Autodesk Fusion 360 part; units mm, degrees
(part 2 of 5)
sketch "Sketch8" plane through (0, 0, 0) normal (0, -1, 0) x (1, 0, 0)
  line L0 (30.55, -4) -> (30.55, 20)
  line L1 (30.55, 20) -> (28.55, 20)
  line L2 (28.55, 20) -> (28.55, -4)
  line L3 (30.55, 20) -> (28.55, 20)
  line L4 (30.55, 36.5) -> (30.55, 20)
  line L5 (-30.55, 20) -> (-28.55, 20)
  line L6 (-30.55, 36.5) -> (-30.55, 20)
  line L7 (28.55, 20) -> (-28.55, 20)
  line L8 (-19.3, 36.5) -> (-19.3, 34.25)
  line L9 (-24.3, 29.25) -> (-26.05, 29.25)
  line L10 (19.3, 36.5) -> (19.3, 34.25)
  line L11 (24.3, 29.25) -> (26.05, 29.25)
  line L12 (-28.55, 26.75) -> (-28.55, 20)
  line L13 (28.55, 26.75) -> (28.55, 20)
  line L14 (-28.05, 39) -> (-21.8, 39)
  line L15 (21.8, 39) -> (28.05, 39)
  arc A0 (30.55, 36.5) -> (28.05, 39) centre (28.05, 36.5) ccw
  arc A1 (-28.05, 39) -> (-30.55, 36.5) centre (-28.05, 36.5) ccw
  arc A2 (21.8, 39) -> (19.3, 36.5) centre (21.8, 36.5) ccw
  arc A3 (28.55, 26.75) -> (26.05, 29.25) centre (26.05, 26.75) ccw
  arc A4 (-26.05, 29.25) -> (-28.55, 26.75) centre (-26.05, 26.75) ccw
  arc A5 (-19.3, 36.5) -> (-21.8, 39) centre (-21.8, 36.5) ccw
  arc A6 (19.3, 34.25) -> (24.3, 29.25) centre (24.3, 34.25) ccw
  arc A7 (-24.3, 29.25) -> (-19.3, 34.25) centre (-24.3, 34.25) ccw
  line L16 (28.55, -4) -> (30.55, -4)
  point P0 (-30.55, 39)
  point P1 (-19.3, 39)
  point P2 (-19.3, 29.25)
  point P3 (-28.55, 29.25)
  point P4 (19.3, 39)
  point P5 (19.3, 29.25)
  point P6 (28.55, 29.25)
  dimension "d41" = 61.1
  dimension "d51" = 9.75
  dimension "d52" = 9.75
  dimension "d53" = 9.25
  dimension "d54" = 9.25
  dimension "d55" = 11.25
  dimension "d56" = 9.25
  dimension "d57" = 2.5
  dimension "d58" = 2.5
  dimension "d59" = 5
  constraint horizontal L3
  constraint vertical L4
  constraint coincident L0.end L1.start
  constraint horizontal L5
  constraint vertical L6
  constraint horizontal L0.end L5.start
  constraint vertical L8
  constraint horizontal L9
  constraint vertical L10
  constraint horizontal L11
  constraint perpendicular L7 L12
  constraint coincident L1.end L2.start
  constraint perpendicular L3 L13
  constraint perpendicular L8 L14
  constraint horizontal P2 P5
  constraint tangent L15 A0
  constraint tangent L4 A0
  constraint coincident P0 L14
  constraint coincident P0 L6
  constraint tangent L14 A1
  constraint tangent L6 A1
  constraint equal A0 A1
  constraint coincident P4 L10
  constraint coincident P4 L15
  constraint tangent L10 A2
  constraint tangent L15 A2
  constraint coincident P6 L11
  constraint coincident P6 L13
  constraint tangent L11 A3
  constraint tangent L13 A3
  constraint equal A2 A3
  constraint coincident P3 L9
  constraint coincident P3 L12
  constraint tangent L9 A4
  constraint tangent L12 A4
  constraint equal A2 A4
  constraint coincident P1 L8
  constraint coincident P1 L14
  constraint tangent L8 A5
  constraint tangent L14 A5
  constraint equal A2 A5
  constraint coincident P5 L11
  constraint coincident P5 L10
  constraint tangent L11 A6
  constraint tangent L10 A6
  constraint coincident P2 L9
  constraint coincident P2 L8
  constraint tangent L9 A7
  constraint tangent L8 A7
  constraint equal A6 A7
  measures "d41" distance of L0.end L5.start
  measures "d51" distance of P1 P2
  measures "d52" distance of P4 P5
  measures "d53" distance of P2 P3
  measures "d54" distance of P5 P6
  measures "d55" distance of P0 P1
  measures "d56" distance of P6 L1.end
  measures "d57" radius of A0
  measures "d58" radius of A2
  measures "d59" radius of A6
extrude "Extrude6" add sketch "Sketch8" against normal blind 20 contours L1 L3 L4 L10 L11 L13 L15 A0 A2 A3 A6 | L5 L6 L8 L9 L12 L14 A1 A4 A5 A7 bodies 1
sketch "Sketch9" plane through (0, 20, 0) normal (0, 1, 0) x (-1, 0, 0)
  arc A0 (-19.3, 36.5) -> (-21.8, 39) centre (-21.8, 36.5) ccw
  line L0 (-21.8, 39) -> (-28.05, 39)
  arc A1 (-28.05, 39) -> (-30.55, 36.5) centre (-28.05, 36.5) ccw
  line L1 (-30.55, 36.5) -> (-30.55, 20)
  line L2 (-30.55, 20) -> (-28.55, 20)
  line L3 (-28.55, 20) -> (-28.55, 26.75)
  arc A2 (-26.05, 29.25) -> (-28.55, 26.75) centre (-26.05, 26.75) ccw
  line L4 (-26.05, 29.25) -> (-24.3, 29.25)
  arc A3 (-24.3, 29.25) -> (-19.3, 34.25) centre (-24.3, 34.25) ccw
  line L5 (-19.3, 34.25) -> (-19.3, 36.5)
  line L6 (30.55, 20) -> (30.55, 36.5)
  point P0 (-24.05, 34.05)
  point P1 (24.05, 34.05)
  dimension "d62" = 6.5
  dimension "d63" = 6.5
  dimension "d64" = 4.95
  constraint horizontal P0 P1
  measures "d62" distance of L1 P0
  measures "d63" distance of P1 L6
  measures "d64" distance of L0 P0
hole "Hole3" at (24.05, 20, 34.05) at (-24.05, 20, 34.05) direction (0, -1, 0) diameter 6.5 depth 12.5 tip angle 180 bodies 1
sketch "Sketch10" plane through (0, 7.5, 0) normal (0, 1, 0) x (-1, 0, 0)
  circle A0 centre (-24.05, 34.05) radius 3.25
  line L0 (-30.55, 36.5) -> (-30.55, 20)
  line L1 (30.55, 20) -> (30.55, 36.5)
  line L2 (-21.8, 39) -> (-28.05, 39)
  point P0 (-24.05, 34.05)
  point P1 (24.05, 34.05)
  dimension "d73" = 6.5
  dimension "d74" = 6.5
  dimension "d75" = 4.95
  constraint horizontal P0 P1
  measures "d73" distance of P0 L0
  measures "d74" distance of P1 L1
  measures "d75" distance of P0 L2
hole "Hole4" at (24.05, 7.5, 34.05) at (-24.05, 7.5, 34.05) direction (0, -1, 0) diameter 3.6 end through all counterbore diameter 6.5 counterbore depth 3 bodies 1
sketch "Sketch11" plane through (30.55, 0, 0) normal (1, 0, 0) x (0, 1, 0)
  line L0 (70.0221, 0) -> (70.0221, 20)
  line L1 (70.0221, 20) -> (20, 20)
  line L2 (20, 20) -> (20, 36.5)
  line L3 (20, 36.5) -> (0, 36.5)
  line L4 (0, 36.5) -> (0, -4)
  line L5 (20, -4) -> (20, -2)
  arc A0 (22, 0) -> (20, -2) centre (22, -2) ccw
  line L6 (22, 0) -> (70.0221, 0)
  arc A1 (8.659, 9.478) -> (8.6579, 10.5518) centre (7.8148, 10.014) ccw
  line L7 (8.659, 9.478) -> (3.8443, 1.8949)
  line L8 (3.8432, 18.1005) -> (8.6579, 10.5518)
  line L9 (0.0001, 36.7902) -> (0.0001, -5.2598)
  arc A2 (3.8432, 18.1005) -> (2.0001, 17.5628) centre (3.0001, 17.5628) ccw
  arc A3 (2.0001, 2.4309) -> (3.8443, 1.8949) centre (3.0001, 2.4309) ccw
  arc A4 (18.0001, 17.5628) -> (16.157, 18.1005) centre (17.0001, 17.5628) ccw
  line L10 (16.088, 20.7084) -> (10.853, 12.3732)
  line L11 (9.1559, 12.3786) -> (3.9952, 20.7138)
  line L12 (3.99, -0.735) -> (9.1549, 7.6441)
  line L13 (15.2412, 22.2402) -> (4.8454, 22.2402)
  line L14 (2.0001, 17.5628) -> (2.0001, 2.4309)
  arc A5 (10.8541, 7.6495) -> (9.1549, 7.6441) centre (10.0062, 7.1193) ccw
  line L15 (20.0001, 40.5402) -> (0.0001, 40.5402)
  arc A6 (3.99, -0.735) -> (4.8412, -2.2598) centre (4.8412, -1.2598) ccw
  line L16 (20.0001, 36.7902) -> (0.0001, 36.7902)
  arc A7 (4.8454, 22.2402) -> (3.9952, 20.7138) centre (4.8454, 21.2402) ccw
  line L17 (15.2454, -2.2598) -> (4.8412, -2.2598)
  line L18 (18.0001, 17.5628) -> (18.0001, 2.4309)
  arc A8 (16.088, 20.7084) -> (15.2412, 22.2402) centre (15.2412, 21.2402) ccw
  line L19 (16.1559, 1.8949) -> (11.3412, 9.478)
  arc A9 (9.1559, 12.3786) -> (10.853, 12.3732) centre (10.0062, 12.9051) ccw
  line L20 (10.8541, 7.6495) -> (16.0933, -0.7296)
  line L21 (11.3423, 10.5518) -> (16.157, 18.1005)
  arc A10 (11.3423, 10.5518) -> (11.3412, 9.478) centre (12.1854, 10.014) ccw
  line L22 (12.713, -5.2598) -> (20.0001, -5.2598)
  arc A11 (16.1559, 1.8949) -> (18.0001, 2.4309) centre (17.0001, 2.4309) ccw
  arc A12 (15.2454, -2.2598) -> (16.0933, -0.7296) centre (15.2454, -1.2598) ccw
  line L23 (0.0001, -5.2598) -> (7.2872, -5.2598)
  line L24 (20.0001, -5.2598) -> (20.0001, 36.7902)
  line L25 (0, -4) -> (20, -4)
  point P0 (9.0001, 11.2652)
  point P1 (11.0001, 11.2652)
  point P2 (18.0001, -1.0098)
  point P3 (2.0001, 20.9902)
  point P4 (10.0001, 10.2652)
  point P5 (10.0062, 10.014)
  point P6 (17.0501, 22.2402)
  point P7 (2.0001, -1.0098)
  point P8 (3.0501, -2.2598)
  point P9 (17.0501, -2.2598)
  point P10 (3.0501, 22.2402)
  point P11 (10.0001, 12.2652)
  point P12 (0.0001, 12.2652)
  point P13 (18.0001, 20.9902)
  dimension "d82" = 2
  dimension "d83" = 2
  dimension "d86" = 22
  dimension "d87" = 22
  dimension "d88" = 14
  dimension "d89" = 14
  dimension "d91" = 3.05
  dimension "d92" = 1
  dimension "d150" = 24.5
  dimension "d151" = 5.7857
  dimension "d152" = 18.3
  constraint perpendicular L13 L24
  constraint perpendicular L13 L14
  constraint coincident P6 L10
  constraint coincident P6 L13
  constraint tangent L10 A8
  constraint tangent L13 A8
  constraint coincident P10 L13
  constraint coincident P10 L11
  constraint tangent L13 A7
  constraint tangent L11 A7
  constraint equal A7 A8
  constraint tangent L11 A9
  constraint tangent L10 A9
  constraint equal A8 A9
  constraint tangent A1 L8
  constraint tangent A1 L7
  constraint equal A1 A8
  constraint coincident P7 L7
  constraint coincident P7 L14
  constraint tangent L7 A3
  constraint tangent A3 L14
  constraint equal A3 A8
  constraint coincident P3 L14
  constraint coincident P3 L8
  constraint tangent A2 L14
  constraint tangent L8 A2
  constraint equal A2 A8
  constraint coincident P8 L12
  constraint coincident P8 L17
  constraint tangent L12 A6
  constraint tangent A6 L17
  constraint equal A6 A8
  constraint coincident P9 L17
  constraint coincident P9 L20
  constraint tangent L17 A12
  constraint tangent L20 A12
  constraint equal A8 A12
  constraint coincident P2 L19
  constraint coincident P2 L18
  constraint tangent L19 A11
  constraint tangent L18 A11
  constraint equal A8 A11
  constraint coincident P13 L21
  constraint coincident P13 L18
  constraint tangent A4 L21
  constraint tangent A4 L18
  constraint equal A4 A8
  constraint tangent L19 A10
  constraint tangent L21 A10
  constraint equal A8 A10
  constraint tangent L12 A5
  constraint tangent A5 L20
  constraint equal A5 A8
  constraint vertical A9.centre A5.centre
  constraint horizontal A10.centre A1.centre
  constraint horizontal A10.centre P5
  constraint vertical A5.centre P5
  measures "d82" distance of L18 L24
  measures "d83" distance of L9 L14
  measures "d86" distance of P2 P13
  measures "d87" distance of P3 P7
  measures "d88" distance of P8 P9
  measures "d89" distance of P6 P10
  measures "d91" distance of P8 L9
  measures "d92" radius of A8
  measures "d150" distance of L13 L17
  measures "d151" distance of A9.centre A5.centre
  measures "d152" distance of L13 L15
extrude "Extrude7" cut sketch "Sketch11" against normal blind 65 contours A1 L7 L8 A2 A3 L14 | A4 L18 L19 L21 A10 A11 | L10 L11 L13 A7 A8 A9 | L12 A5 A6 L17 L20 A12 bodies 1
sketch "Sketch12" plane through (30.55, 0, 0) normal (1, 0, 0) x (0, 1, 0)
  line L0 (16.1559, 1.8949) -> (11.3412, 9.478)
  arc A0 (11.3423, 10.5518) -> (11.3412, 9.478) centre (12.1854, 10.014) ccw
  line L1 (11.3423, 10.5518) -> (16.157, 18.1005)
  arc A1 (18.0001, 17.5628) -> (16.157, 18.1005) centre (17.0001, 17.5628) ccw
  line L2 (18.0001, 17.5628) -> (18.0001, 2.4309)
  arc A2 (16.1559, 1.8949) -> (18.0001, 2.4309) centre (17.0001, 2.4309) ccw
  line L3 (15.2454, -2.2598) -> (4.8412, -2.2598)
  arc A3 (3.99, -0.735) -> (4.8412, -2.2598) centre (4.8412, -1.2598) ccw
  line L4 (3.99, -0.735) -> (9.1549, 7.6441)
  arc A4 (10.8541, 7.6495) -> (9.1549, 7.6441) centre (10.0062, 7.1193) ccw
  line L5 (10.8541, 7.6495) -> (16.0933, -0.7296)
  arc A5 (15.2454, -2.2598) -> (16.0933, -0.7296) centre (15.2454, -1.2598) ccw
  line L6 (4.8454, 22.2402) -> (15.2412, 22.2402)
  arc A6 (16.088, 20.7084) -> (15.2412, 22.2402) centre (15.2412, 21.2402) ccw
  line L7 (16.088, 20.7084) -> (10.853, 12.3732)
  arc A7 (9.1559, 12.3786) -> (10.853, 12.3732) centre (10.0062, 12.9051) ccw
  line L8 (9.1559, 12.3786) -> (3.9952, 20.7138)
  arc A8 (4.8454, 22.2402) -> (3.9952, 20.7138) centre (4.8454, 21.2402) ccw
  line L9 (2.0001, 2.4309) -> (2.0001, 17.5628)
  arc A9 (3.8432, 18.1005) -> (2.0001, 17.5628) centre (3.0001, 17.5628) ccw
  line L10 (3.8432, 18.1005) -> (8.6579, 10.5518)
  arc A10 (8.659, 9.478) -> (8.6579, 10.5518) centre (7.8148, 10.014) ccw
  line L11 (8.659, 9.478) -> (3.8443, 1.8949)
  arc A11 (2.0001, 2.4309) -> (3.8443, 1.8949) centre (3.0001, 2.4309) ccw
  line L12 (70.0221, 0) -> (70.0221, 20)
  line L13 (70.0221, 20) -> (20, 20)
  line L14 (20, 20) -> (20, 36.5)
  line L15 (20, 36.5) -> (0, 36.5)
  line L16 (0, 36.5) -> (0, -4)
  line L17 (20, -4) -> (20, -2)
  arc A12 (22, 0) -> (20, -2) centre (22, -2) ccw
  line L18 (22, 0) -> (70.0221, 0)
  line L19 (27.57, 18) -> (62.43, 18)
  line L20 (68, 14.6743) -> (68, 5.3257)
  line L21 (62.43, 2) -> (27.57, 2)
  line L22 (22, 5.3257) -> (22, 14.6743)
  line L23 (27.4327, 17.0192) -> (44.7253, 12.0785)
  line L24 (45.2747, 12.0785) -> (62.5673, 17.0192)
  line L25 (66.7253, 15.6358) -> (48.6827, 10.4808)
  line L26 (48.6827, 9.5192) -> (66.7253, 4.3642)
  line L27 (62.5673, 2.9808) -> (45.2747, 7.9215)
  line L28 (44.7253, 7.9215) -> (27.4327, 2.9808)
  line L29 (23.2747, 4.3642) -> (41.3173, 9.5192)
  line L30 (41.3173, 10.4808) -> (23.2747, 15.6358)
  arc A13 (23.2747, 15.6358) -> (22, 14.6743) centre (23, 14.6743) ccw
  arc A14 (22, 5.3257) -> (23.2747, 4.3642) centre (23, 5.3257) ccw
  arc A15 (66.7253, 4.3642) -> (68, 5.3257) centre (67, 5.3257) ccw
  arc A16 (68, 14.6743) -> (66.7253, 15.6358) centre (67, 14.6743) ccw
  arc A17 (41.3173, 9.5192) -> (41.3173, 10.4808) centre (41.18, 10) ccw
  arc A18 (48.6827, 10.4808) -> (48.6827, 9.5192) centre (48.82, 10) ccw
  arc A19 (27.4327, 2.9808) -> (27.57, 2) centre (27.57, 2.5) ccw
  arc A20 (62.43, 2) -> (62.5673, 2.9808) centre (62.43, 2.5) ccw
  arc A21 (62.5673, 17.0192) -> (62.43, 18) centre (62.43, 17.5) ccw
  arc A22 (27.57, 18) -> (27.4327, 17.0192) centre (27.57, 17.5) ccw
  arc A23 (44.7253, 12.0785) -> (45.2747, 12.0785) centre (45, 13.04) ccw
  arc A24 (45.2747, 7.9215) -> (44.7253, 7.9215) centre (45, 6.96) ccw
  line L31 (0, -4) -> (20, -4)
  point P0 (24, 18)
  point P1 (22, 16)
  point P2 (22, 4)
  point P3 (24, 2)
  point P4 (66, 18)
  point P5 (68, 16)
  point P6 (68, 4)
  point P7 (66, 2)
  point P8 (45, 10)
  point P9 (45, 12)
  point P10 (43, 10)
  point P11 (45, 8)
  point P12 (47, 10)
  dimension "d95" = 1
  dimension "d96" = 0.5
  dimension "d97" = 0.5
  dimension "d98" = 1
  constraint horizontal L19
  constraint vertical L20
  constraint horizontal L21
  constraint vertical L22
  constraint coincident L19 P0
  constraint coincident L22 P1
  constraint coincident L22 P2
  constraint coincident L21 P3
  constraint coincident L19 P4
  constraint coincident L20 P5
  constraint coincident L20 P6
  constraint coincident L21 P7
  constraint parallel L24 L25
  constraint parallel L23 L26
  constraint parallel L26 L27
  constraint parallel L25 L28
  constraint parallel L28 L29
  constraint parallel L27 L30
  constraint tangent L30 A13
  constraint tangent L22 A13
  constraint tangent L29 A14
  constraint tangent L22 A14
  constraint equal A13 A14
  constraint tangent L26 A15
  constraint tangent L20 A15
  constraint equal A13 A15
  constraint tangent L25 A16
  constraint tangent L20 A16
  constraint equal A13 A16
  constraint tangent L30 A17
  constraint tangent L29 A17
  constraint tangent L26 A18
  constraint tangent L25 A18
  constraint equal A17 A18
  constraint tangent L28 A19
  constraint tangent L21 A19
  constraint tangent L21 A20
  constraint tangent L27 A20
  constraint equal A19 A20
  constraint tangent L24 A21
  constraint tangent L19 A21
  constraint equal A19 A21
  constraint tangent L23 A22
  constraint tangent L19 A22
  constraint equal A19 A22
  constraint tangent L23 A23
  constraint tangent L24 A23
  constraint tangent L28 A24
  constraint tangent L27 A24
  constraint equal A23 A24
  measures "d95" radius of A13
  measures "d96" radius of A17
  measures "d97" radius of A19
  measures "d98" radius of A23
extrude "Extrude8" cut sketch "Sketch12" against normal blind 65 contours L19 L23 L24 A21 A22 A23 | L20 L25 L26 A15 A16 A18 | L21 L27 L28 A19 A20 A24 | L22 L29 L30 A13 A14 A17 bodies 1
sketch "Sketch15" plane through (0, 0, 0) normal (0, -1, 0) x (1, 0, 0)
  circle A0 centre (-24.05, 34.05) radius 1.8
  line L0 (-28.55, -4) -> (-28.55, 26.75)
  arc A1 (-26.05, 29.25) -> (-28.55, 26.75) centre (-26.05, 26.75) ccw
  line L1 (-26.05, 29.25) -> (-24.3, 29.25)
  arc A2 (-24.3, 29.25) -> (-19.3, 34.25) centre (-24.3, 34.25) ccw
  line L2 (-19.3, 34.25) -> (-19.3, 36.5)
  arc A3 (-19.3, 36.5) -> (-21.8, 39) centre (-21.8, 36.5) ccw
  line L3 (-21.8, 39) -> (-28.05, 39)
  arc A4 (-28.05, 39) -> (-30.55, 36.5) centre (-28.05, 36.5) ccw
  line L4 (-30.55, 36.5) -> (-30.55, -4)
  line L5 (-21.4029, 18) -> (21.4029, 18)
  line L6 (26.55, 15.2137) -> (26.55, 4.7863)
  line L7 (21.4029, 2) -> (-21.4029, 2)
  line L8 (-26.55, 4.7863) -> (-26.55, 15.2137)
  line L9 (28.55, 0) -> (-28.55, 0)
  line L10 (28.55, 20) -> (-28.55, 20)
  line L11 (28.55, -4) -> (28.55, 26.75)
  line L12 (-21.527, 2.9844) -> (-1.241, 8.182)
  line L13 (1.241, 8.182) -> (21.527, 2.9844)
  line L14 (25.3035, 3.8171) -> (3.8571, 9.2732)
  line L15 (3.8571, 10.7268) -> (25.3035, 16.1829)
  line L16 (21.527, 17.0156) -> (1.241, 11.818)
  line L17 (-1.241, 11.818) -> (-21.527, 17.0156)
  line L18 (-25.3035, 16.1829) -> (-3.8571, 10.7268)
  line L19 (-3.8571, 9.2732) -> (-25.3035, 3.8171)
  arc A5 (-25.3035, 16.1829) -> (-26.55, 15.2137) centre (-25.55, 15.2137) ccw
  arc A6 (-26.55, 4.7863) -> (-25.3035, 3.8171) centre (-25.55, 4.7863) ccw
  arc A7 (25.3035, 3.8171) -> (26.55, 4.7863) centre (25.55, 4.7863) ccw
  arc A8 (26.55, 15.2137) -> (25.3035, 16.1829) centre (25.55, 15.2137) ccw
  arc A9 (-3.8571, 9.2732) -> (-3.8571, 10.7268) centre (-4.042, 10) ccw
  arc A10 (3.8571, 10.7268) -> (3.8571, 9.2732) centre (4.042, 10) ccw
  arc A11 (-21.527, 2.9844) -> (-21.4029, 2) centre (-21.4029, 2.5) ccw
  arc A12 (21.4029, 2) -> (21.527, 2.9844) centre (21.4029, 2.5) ccw
  arc A13 (21.527, 17.0156) -> (21.4029, 18) centre (21.4029, 17.5) ccw
  arc A14 (-21.4029, 18) -> (-21.527, 17.0156) centre (-21.4029, 17.5) ccw
  arc A15 (-1.241, 11.818) -> (1.241, 11.818) centre (0, 16.6615) ccw
  arc A16 (1.241, 8.182) -> (-1.241, 8.182) centre (0, 3.3385) ccw
  line L20 (-30.55, -4) -> (-28.55, -4)
  point P0 (-26.55, 18)
  point P1 (26.55, 18)
  point P2 (26.55, 2)
  point P3 (-25.05, 18)
  point P4 (-25.05, 2)
  point P5 (25.05, 18)
  point P6 (25.05, 2)
  point P7 (0, 10)
  point P8 (-26.55, 16.5)
  point P9 (-26.55, 3.5)
  point P10 (26.55, 16.5)
  point P11 (26.55, 3.5)
  point P12 (0, 8.5)
  point P13 (-1, 10)
  point P14 (0, 11.5)
  point P15 (1, 10)
  dimension "d102" = 2
  dimension "d103" = 2
  dimension "d104" = 2
  dimension "d105" = 2
  dimension "d106" = 1.5
  dimension "d107" = 1.5
  dimension "d108" = 1.5
  dimension "d109" = 1.5
  dimension "d110" = 26.55
  dimension "d112" = 1
  dimension "d113" = 0.75
  dimension "d114" = 0.5
  dimension "d115" = 3
  dimension "d117" = 1.5
  dimension "d118" = 5
  constraint horizontal L5
  constraint vertical L6
  constraint horizontal L7
  constraint vertical L8
  constraint coincident L5 P3
  constraint coincident L7 P4
  constraint coincident L5 P5
  constraint coincident L7 P6
  constraint coincident L8 P8
  constraint coincident L8 P9
  constraint coincident L6 P10
  constraint coincident L6 P11
  constraint vertical P3 P4
  constraint horizontal P8 P10
  constraint horizontal P9 P11
  constraint vertical P5 P6
  constraint coincident P0 L8
  constraint tangent L18 A5
  constraint tangent L8 A5
  constraint tangent L19 A6
  constraint tangent L8 A6
  constraint equal A5 A6
  constraint coincident P2 L6
  constraint tangent L14 A7
  constraint tangent L6 A7
  constraint equal A5 A7
  constraint coincident P1 L6
  constraint tangent L6 A8
  constraint tangent L15 A8
  constraint equal A5 A8
  constraint tangent L19 A9
  constraint tangent L18 A9
  constraint tangent L14 A10
  constraint tangent L15 A10
  constraint equal A9 A10
  constraint tangent L12 A11
  constraint tangent L7 A11
  constraint coincident P2 L7
  constraint tangent L13 A12
  constraint tangent L7 A12
  constraint equal A11 A12
  constraint coincident P1 L5
  constraint tangent L16 A13
  constraint tangent L5 A13
  constraint equal A11 A13
  constraint coincident P0 L5
  constraint tangent L17 A14
  constraint tangent L5 A14
  constraint equal A11 A14
  constraint vertical P12 P14
  constraint horizontal A9.centre A10.centre
  constraint vertical P7 P12
  constraint horizontal P7 A10.centre
  constraint tangent L17 A15
  constraint tangent L16 A15
  constraint tangent L12 A16
  constraint tangent L13 A16
  constraint equal A15 A16
  measures "d102" distance of L0 L8
  measures "d103" distance of L7 L9
  measures "d104" distance of L5 L10
  measures "d105" distance of L6 L11
  measures "d106" distance of P0 P3
  measures "d107" distance of P0 P8
  measures "d108" distance of P1 P5
  measures "d109" distance of P2 P11
  measures "d110" horizontal distance of P0 P7
  measures "d112" radius of A5
  measures "d113" radius of A9
  measures "d114" radius of A11
  measures "d115" distance of P12 P14
  measures "d117" distance of P7 P12
  measures "d118" radius of A15
extrude "Extrude9" cut sketch "Sketch15" against normal blind 80 contours L5 L16 L17 A13 A14 A15 | L6 L14 L15 A7 A8 A10 | L7 L12 L13 A11 A12 A16 | L8 L18 L19 A5 A6 A9 bodies 1
sketch "Sketch17" plane through (0, 0, 0) normal (0, -1, 0) x (1, 0, 0)
  circle A0 centre (24.05, 34.05) radius 1.8
  line L0 (30.55, -4) -> (30.55, 36.5)
  arc A1 (30.55, 36.5) -> (28.05, 39) centre (28.05, 36.5) ccw
  line L1 (28.05, 39) -> (21.8, 39)
  arc A2 (21.8, 39) -> (19.3, 36.5) centre (21.8, 36.5) ccw
  line L2 (19.3, 36.5) -> (19.3, 34.25)
  arc A3 (19.3, 34.25) -> (24.3, 29.25) centre (24.3, 34.25) ccw
  line L3 (24.3, 29.25) -> (26.05, 29.25)
  arc A4 (28.55, 26.75) -> (26.05, 29.25) centre (26.05, 26.75) ccw
  line L4 (28.55, 26.75) -> (28.55, -4)
  line L5 (28.55, -4) -> (30.55, -4)
  line L6 (28.55, -4) -> (30.55, -4)
  line L7 (30.55, -4) -> (30.55, -18.55)
  line L8 (30.55, -18.55) -> (28.55, -18.55)
  line L9 (28.55, -18.55) -> (28.55, -4)
  line L10 (-28.55, -4) -> (-30.55, -4)
  line L11 (-30.55, -4) -> (-30.55, -18.55)
  line L12 (-30.55, -18.55) -> (-28.55, -18.55)
  line L13 (-28.55, -18.55) -> (-28.55, -4)
  line L14 (-30.55, -18.55) -> (-40.55, -18.55)
  line L15 (-40.55, -18.55) -> (-40.55, -16.05)
  line L16 (-40.55, -16.05) -> (-30.55, -16.05)
  line L17 (-30.55, -16.05) -> (-30.55, -18.55)
  line L18 (30.55, -18.55) -> (40.55, -18.55)
  line L19 (40.55, -18.55) -> (40.55, -16.05)
  line L20 (40.55, -16.05) -> (30.55, -16.05)
  line L21 (30.55, -16.05) -> (30.55, -18.55)
  dimension "d128" = 57.55
  dimension "d129" = 57.1
  dimension "d130" = 2
  dimension "d131" = 2
  dimension "d132" = 2.5
  dimension "d133" = 10
  dimension "d134" = 10
  dimension "d135" = 2.5
  constraint horizontal L6
  constraint vertical L7
  constraint horizontal L8
  constraint vertical L9
  constraint coincident L4.end L5.start
  constraint horizontal L10
  constraint vertical L11
  constraint horizontal L12
  constraint vertical L13
  constraint horizontal L7.end L12.end
  constraint horizontal L4.end L10.start
  constraint horizontal L14
  constraint vertical L15
  constraint horizontal L16
  constraint vertical L17
  constraint horizontal L18
  constraint vertical L19
  constraint horizontal L20
  constraint vertical L21
  measures "d128" distance of L1 L8
  measures "d129" distance of L9 L13
  measures "d130" distance of L11 L13
  measures "d131" distance of L7 L9
  measures "d132" distance of L18 L20
  measures "d133" distance of L7 L19
  measures "d134" distance of L15 L17
  measures "d135" distance of L14 L16
extrude "Extrude11" add sketch "Sketch17" against normal blind 20 contours L5 L6 L7 L8 L9 L21 | L7 L18 L19 L20 L21 | L10 L11 L12 L13 L17 | L11 L14 L15 L16 L17 bodies 1
fillet "Fillet3" radius 2 2 edges at (40.55, 20, -17.3) (-40.55, 20, -17.3) on bodies 1
fillet "Fillet4" radius 2 2 edges at (-29.55, 20, 20) (29.55, 20, 20) on bodies 1
extrude "Extrude12" cut 2 faces at (-32.55, 12.6667, -18.55) (32.55, 12.6667, -18.55) along direction (0, 0, 1) blind 0.05 on bodies 1 bodies 1
extrude "Extrude13" add 2 faces at (33.8833, 12.6667, -16.05) (-33.8833, 12.6667, -16.05) along direction (0, 0, 1) blind 7.55 on bodies 1 bodies 1
sketch "Sketch19" plane through (0, 0, -8.5) normal (0, 0, 1) x (-1, 0, 0)
  arc A0 (-40.55, -18) -> (-38.55, -20) centre (-38.55, -18) ccw
  line L0 (-38.55, -20) -> (-30.55, -20)
  line L1 (-30.55, -20) -> (-30.55, 0)
  line L2 (-30.55, 0) -> (-40.55, 0)
  line L3 (-40.55, 0) -> (-40.55, -18)
  point P0 (-34.75, -10)
  point P1 (34.75, -10)
  dimension "d159" = 69.5
  dimension "d160" = 5.8
  dimension "d161" = 10
  constraint horizontal P0 P1
  measures "d159" distance of P0 P1
  measures "d160" distance of L3 P0
  measures "d161" distance of L2 P0
hole "Hole6" at (-34.75, 10, -8.5) at (34.75, 10, -8.5) direction (0, 0, -1) diameter 5.3 depth 10 tip angle 118 counterbore diameter 10 counterbore depth 5 bodies 1
sketch "Sketch20" plane through (0, 0, -8.5) normal (0, 0, 1) x (-1, 0, 0)
  arc A0 (-30.55, -7.2871) -> (-30.55, -12.7129) centre (-34.75, -10) ccw
  line L0 (-30.55, -7.2871) -> (-30.55, 0)
  line L1 (-30.55, 0) -> (-40.55, 0)
  line L2 (-40.55, 0) -> (-40.55, -18)
  arc A1 (-40.55, -18) -> (-38.55, -20) centre (-38.55, -18) ccw
  line L3 (-38.55, -20) -> (-30.55, -20)
  line L4 (-30.55, -20) -> (-30.55, -12.7129)
  circle A2 centre (-34.75, -10) radius 5
  circle A3 centre (34.75, -10) radius 5
  dimension "d167" = 10
  dimension "d168" = 10
  dimension "d169" = 69.5
  constraint concentric A0 A2
  constraint horizontal A0.centre A3.centre
  measures "d167" diameter of A2
  measures "d168" diameter of A3
  measures "d169" distance of A0.centre A3.centre
extrude "Extrude14" cut sketch "Sketch20" along normal blind 7 contours A0 A2 | A3 bodies 1
equation "d6 = ( 57.1 / 2 ) * 1 mm"
equation "d64 = 6.5 mm - 1.55 mm"
equation "d75 = 6.5 mm - 1.55 mm"
equation "d110 = ( 53.1 / 2 ) * 1 mm"
equation "d157 = 10 mm - 2.45 mm"

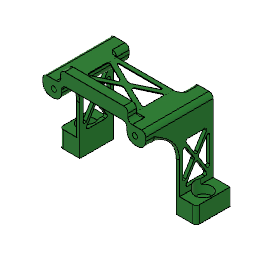
design "LGR RM Front Holder (Goalie)"
Autodesk Fusion 360 part; units mm, degrees
sketch "Sketch1" plane through (0, 0, 0) normal (0, 0, 1) x (1, 0, 0)
  line L0 (28.55, 26.275) -> (30.55, 26.275)
  line L1 (30.55, 26.275) -> (30.55, -26.275)
  line L2 (30.55, -26.275) -> (28.55, -26.275)
  line L3 (28.55, -26.275) -> (28.55, 26.275)
  line L4 (-28.55, -26.275) -> (-30.55, -26.275)
  line L5 (-28.55, 26.275) -> (-28.55, -26.275)
  line L6 (-30.55, -26.275) -> (-30.55, 26.275)
  line L7 (-30.55, 26.275) -> (-28.55, 26.275)
  line L8 (-30.55, 26.275) -> (30.55, 26.275)
  line L9 (30.55, 26.275) -> (30.55, 28.275)
  line L10 (30.55, 28.275) -> (-30.55, 28.275)
  line L11 (-30.55, 28.275) -> (-30.55, 26.275)
  dimension "d1" = 2
  dimension "d2" = 52.55
  dimension "d4" = 26.275
  dimension "d5" = 2
  dimension "d6" = 52.55
  dimension "d7" = 57.1
  dimension "d8" = 28.55
  dimension "d9" = 2
  constraint horizontal L0
  constraint vertical L1
  constraint horizontal L2
  constraint vertical L3
  constraint horizontal L7
  constraint vertical L5
  constraint horizontal L4
  constraint vertical L6
  constraint horizontal L2.end L4.start
  constraint horizontal L8
  constraint vertical L9
  constraint horizontal L10
  constraint vertical L11
  constraint vertical L0.end L9.end
  measures "d1" distance of L1 L3
  measures "d2" distance of L0 L2
  measures "d4" distance of origin L0
  measures "d5" distance of L5 L6
  measures "d6" distance of L4 L7
  measures "d7" distance of L3 L5
  measures "d8" distance of origin L5
  measures "d9" distance of L8 L10
extrude "Extrude1" add sketch "Sketch1" along normal blind 20
sketch "Sketch2" plane through (0, 0, 20) normal (0, 0, 1) x (-1, 0, 0)
  line L0 (-30.55, 26.275) -> (-30.55, -28.275)
  line L1 (-30.55, -28.275) -> (30.55, -28.275)
  line L2 (30.55, -28.275) -> (30.55, 26.275)
  line L3 (30.55, 26.275) -> (28.55, 26.275)
  line L4 (28.55, 26.275) -> (28.55, -26.275)
  line L5 (28.55, -26.275) -> (-28.55, -26.275)
  line L6 (-28.55, -26.275) -> (-28.55, 26.275)
  line L7 (-28.55, 26.275) -> (-30.55, 26.275)
  line L8 (-30.55, 26.275) -> (-40.55, 26.275)
  line L9 (-40.55, 26.275) -> (-40.55, 16.275)
  line L10 (-40.55, 16.275) -> (-30.55, 16.275)
  line L11 (-30.55, 16.275) -> (-30.55, 26.275)
  line L12 (30.55, 26.275) -> (40.55, 26.275)
  line L13 (40.55, 26.275) -> (40.55, 16.275)
  line L14 (40.55, 16.275) -> (30.55, 16.275)
  line L15 (30.55, 16.275) -> (30.55, 26.275)
  dimension "d12" = 10
  dimension "d13" = 10
  dimension "d14" = 10
  dimension "d15" = 10
  constraint horizontal L8
  constraint vertical L9
  constraint horizontal L10
  constraint vertical L11
  constraint coincident L0.start L7.end
  constraint horizontal L12
  constraint vertical L13
  constraint horizontal L14
  constraint vertical L15
  constraint coincident L2.end L3.start
  measures "d12" distance of L8 L10
  measures "d13" distance of L9 L11
  measures "d14" distance of L12 L14
  measures "d15" distance of L13 L15
extrude "Extrude2" add sketch "Sketch2" against normal blind 20 contours L0 L8 L9 L10 L11 | L2 L12 L13 L14 L15
fillet "Fillet1" radius 2 2 edges at (40.55, -21.275, 0) (-40.55, -21.275, 0)
sketch "Sketch3" plane through (0, -16.275, 0) normal (0, 1, 0) x (-1, 0, 0)
  arc A0 (38.55, 0) -> (40.55, 2) centre (38.55, 2) ccw
  line L0 (40.55, 2) -> (40.55, 20)
  line L1 (40.55, 20) -> (30.55, 20)
  line L2 (30.55, 20) -> (30.55, 0)
  line L3 (30.55, 0) -> (38.55, 0)
  point P0 (34.75, 10)
  point P1 (-34.75, 10)
  dimension "d20" = 5.8
  dimension "d21" = 10
  dimension "d22" = 69.5
  constraint horizontal P0 P1
  measures "d20" distance of L0 P0
  measures "d21" distance of L3 P0
  measures "d22" distance of P0 P1
hole "Hole1" at (-34.75, -16.275, 10) at (34.75, -16.275, 10) direction (0, -1, 0) diameter 5.3 end through all counterbore diameter 10 counterbore depth 5
sketch "Sketch4" plane through (0, -16.275, 0) normal (0, 1, 0) x (-1, 0, 0)
  arc A0 (30.55, 7.2871) -> (30.55, 12.7129) centre (34.75, 10) ccw
  line L0 (30.55, 7.2871) -> (30.55, 0)
  line L1 (30.55, 0) -> (38.55, 0)
  arc A1 (38.55, 0) -> (40.55, 2) centre (38.55, 2) ccw
  line L2 (40.55, 2) -> (40.55, 20)
  line L3 (40.55, 20) -> (30.55, 20)
  line L4 (30.55, 20) -> (30.55, 12.7129)
  circle A2 centre (34.75, 10) radius 5
  circle A3 centre (-34.75, 10) radius 5
  dimension "d28" = 10
  dimension "d29" = 69.5
  constraint concentric A0 A2
  constraint coincident A0.end A2
  constraint horizontal A0.centre A3.centre
  measures "d28" diameter of A3
  measures "d29" distance of A0.centre A3.centre
extrude "Extrude3" cut sketch "Sketch4" along normal blind 7 contours A0 A2 | A3
sketch "Sketch5" plane through (0, 28.275, 0) normal (0, 1, 0) x (-1, 0, 0)
  line L0 (-30.55, 0) -> (30.55, 0)
  line L1 (30.55, 0) -> (30.55, 20)
  line L2 (30.55, 20) -> (-30.55, 20)
  line L3 (-30.55, 20) -> (-30.55, 0)
  line L4 (-20, 20) -> (20, 20)
  line L5 (20, 20) -> (20, 0)
  line L6 (20, 0) -> (-20, 0)
  line L7 (-20, 0) -> (-20, 20)
  dimension "d32" = 40
  dimension "d96" = 20
  constraint horizontal L4
  constraint vertical L5
  constraint horizontal L6
  constraint vertical L7
  constraint coincident L0 L5.end
  constraint coincident L2 L4.start
  measures "d32" distance of L5 L7
  measures "d96" distance of origin L7
extrude "Extrude4" add sketch "Sketch5" along normal blind 10 contours L0 L2 L4 L5 L6 L7
sketch "Sketch6" plane through (0, 0, 0) normal (0, 0, -1) x (1, 0, 0)
  line L0 (20, -38.275) -> (20, -28.275)
  line L1 (-30.55, -28.275) -> (-20, -28.275)
  line L2 (30.55, -28.275) -> (30.55, 16.275)
  line L3 (30.55, 16.275) -> (38.55, 16.275)
  line L4 (38.55, 16.275) -> (38.55, 26.275)
  line L5 (38.55, 26.275) -> (28.55, 26.275)
  line L6 (28.55, 26.275) -> (28.55, -26.275)
  line L7 (28.55, -26.275) -> (-28.55, -26.275)
  line L8 (-28.55, -26.275) -> (-28.55, 26.275)
  line L9 (-28.55, 26.275) -> (-38.55, 26.275)
  line L10 (-38.55, 26.275) -> (-38.55, 16.275)
  line L11 (-38.55, 16.275) -> (-30.55, 16.275)
  line L12 (-30.55, 16.275) -> (-30.55, -28.275)
  line L13 (-20, -28.275) -> (-20, -38.275)
  line L14 (-20, -38.275) -> (20, -38.275)
  line L15 (-28.55, -26.275) -> (-19.3, -26.275)
  line L16 (-19.3, -23.775) -> (-19.3, -22.025)
  line L17 (-24.3, -17.025) -> (-26.05, -17.025)
  line L18 (-28.55, -17.025) -> (-28.55, -26.275)
  line L19 (28.55, -26.275) -> (19.3, -26.275)
  line L20 (19.3, -23.775) -> (19.3, -22.025)
  line L21 (24.3, -17.025) -> (26.05, -17.025)
  line L22 (28.55, -17.025) -> (28.55, -26.275)
  arc A0 (-19.3, -22.025) -> (-24.3, -17.025) centre (-24.3, -22.025) ccw
  arc A1 (24.3, -17.025) -> (19.3, -22.025) centre (24.3, -22.025) ccw
  line L23 (28.55, -14.525) -> (28.55, -10)
  line L24 (-28.55, -14.525) -> (-28.55, -10)
  arc A2 (26.05, -17.025) -> (28.55, -14.525) centre (26.05, -14.525) ccw
  arc A3 (-28.55, -14.525) -> (-26.05, -17.025) centre (-26.05, -14.525) ccw
  line L25 (16.8, -26.275) -> (13, -26.275)
  line L26 (-16.8, -26.275) -> (-13, -26.275)
  arc A4 (16.8, -26.275) -> (19.3, -23.775) centre (16.8, -23.775) ccw
  arc A5 (-19.3, -23.775) -> (-16.8, -26.275) centre (-16.8, -23.775) ccw
  line L27 (20, -28.275) -> (30.55, -28.275)
  dimension "d38" = 9.25
  dimension "d39" = 9.25
  dimension "d40" = 9.25
  dimension "d41" = 9.25
  dimension "d42" = 5
  dimension "d43" = 5
  dimension "d44" = 2.5
  dimension "d45" = 2.5
  dimension "d46" = 2.5
  dimension "d47" = 2.5
  constraint horizontal L15
  constraint vertical L16
  constraint horizontal L17
  constraint vertical L18
  constraint coincident L7.end L8.start
  constraint horizontal L19
  constraint vertical L20
  constraint horizontal L21
  constraint vertical L22
  constraint coincident L6.end L7.start
  constraint tangent L17 A0
  constraint tangent L16 A0
  constraint tangent L21 A1
  constraint tangent L20 A1
  constraint coincident L6 L23.end
  constraint coincident L8 L24.end
  constraint coincident L22.start L21
  constraint coincident L22.start L23
  constraint tangent L21 A2
  constraint tangent L23 A2
  constraint coincident L18.start L24
  constraint coincident L18.start L17
  constraint tangent L24 A3
  constraint tangent L17 A3
  constraint coincident L7 L25.end
  constraint coincident L7 L26.end
  constraint coincident L19.end L25
  constraint coincident L19.end L20
  constraint tangent L25 A4
  constraint tangent L20 A4
  constraint coincident L15.end L26
  constraint coincident L15.end L16
  constraint tangent L26 A5
  constraint tangent L16 A5
  measures "d38" distance of L16 L18
  measures "d39" distance of L15 L17
  measures "d40" distance of L20 L22
  measures "d41" distance of L19 L21
  measures "d42" radius of A0
  measures "d43" radius of A1
  measures "d44" radius of A2
  measures "d45" radius of A3
  measures "d46" radius of A4
  measures "d47" radius of A5
extrude "Extrude5" add sketch "Sketch6" against normal blind 20 contours L6 L7 L19 L20 L21 L22 A1 A2 A4 | L7 L8 L15 L16 L17 L18 A0 A3 A5
sketch "Sketch7" plane through (0, 0, 20) normal (0, 0, 1) x (-1, 0, 0)
  line L0 (-30.55, -28.275) -> (-20, -28.275)
  line L1 (-20, -28.275) -> (20, -28.275)
  line L2 (30.55, -28.275) -> (30.55, 16.275)
  line L3 (30.55, 16.275) -> (40.55, 16.275)
  line L4 (40.55, 16.275) -> (40.55, 26.275)
  line L5 (40.55, 26.275) -> (28.55, 26.275)
  line L6 (28.55, 26.275) -> (28.55, -14.525)
  arc A0 (26.05, -17.025) -> (28.55, -14.525) centre (26.05, -14.525) ccw
  line L7 (26.05, -17.025) -> (24.3, -17.025)
  arc A1 (24.3, -17.025) -> (19.3, -22.025) centre (24.3, -22.025) ccw
  line L8 (19.3, -22.025) -> (19.3, -23.775)
  arc A2 (16.8, -26.275) -> (19.3, -23.775) centre (16.8, -23.775) ccw
  line L9 (16.8, -26.275) -> (-16.8, -26.275)
  arc A3 (-19.3, -23.775) -> (-16.8, -26.275) centre (-16.8, -23.775) ccw
  line L10 (-19.3, -23.775) -> (-19.3, -22.025)
  arc A4 (-19.3, -22.025) -> (-24.3, -17.025) centre (-24.3, -22.025) ccw
  line L11 (-24.3, -17.025) -> (-26.05, -17.025)
  arc A5 (-28.55, -14.525) -> (-26.05, -17.025) centre (-26.05, -14.525) ccw
  line L12 (-28.55, -14.525) -> (-28.55, 26.275)
  line L13 (-28.55, 26.275) -> (-40.55, 26.275)
  line L14 (-40.55, 26.275) -> (-40.55, 16.275)
  line L15 (-40.55, 16.275) -> (-30.55, 16.275)
  line L16 (-30.55, 16.275) -> (-30.55, -28.275)
  line L17 (20, -28.275) -> (30.55, -28.275)
  point P0 (24.05, -21.775)
  point P1 (-24.05, -21.775)
  dimension "d52" = 6.5
  dimension "d54" = 6.5
  constraint horizontal P0 P1
  measures "d52" distance of L2 P0
  measures "d54" distance of L16 P1
hole "Hole2" at (-24.05, 21.775, 20) at (24.05, 21.775, 20) direction (0, 0, -1) diameter 3 end through all
sketch "Sketch10" plane through (-30.55, 0, 0) normal (-1, 0, 0) x (0, -1, 0)
  line L0 (-28.275, 0) -> (16.275, 0)
  line L1 (16.275, 0) -> (16.275, 7.2871)
  line L2 (16.275, 7.2871) -> (9.275, 7.2871)
  line L3 (9.275, 7.2871) -> (9.275, 12.7129)
  line L4 (9.275, 12.7129) -> (16.275, 12.7129)
  line L5 (16.275, 12.7129) -> (16.275, 20)
  line L6 (16.275, 20) -> (-28.275, 20)
  line L7 (-11.225, 15.2411) -> (-11.225, 4.8453)
  line L8 (13.275, 15.2453) -> (13.275, 4.8411)
  line L9 (-28.275, 20) -> (-28.275, 0)
  line L10 (-6.5475, 18) -> (8.5844, 18)
  line L11 (-6.5475, 2) -> (8.5844, 2)
  line L12 (-7.0853, 3.8431) -> (0.4635, 8.6578)
  line L13 (1.5372, 8.6589) -> (9.1204, 3.8442)
  line L14 (11.7503, 3.9899) -> (3.3712, 9.1548)
  line L15 (3.3657, 10.854) -> (11.7448, 16.0932)
  line L16 (9.1204, 16.1558) -> (1.5372, 11.3411)
  line L17 (0.4635, 11.3422) -> (-7.0853, 16.1569)
  line L18 (-9.6931, 16.0879) -> (-1.358, 10.8529)
  line L19 (-1.3634, 9.1558) -> (-9.6986, 3.9951)
  arc A0 (-9.6931, 16.0879) -> (-11.225, 15.2411) centre (-10.225, 15.2411) ccw
  arc A1 (-11.225, 4.8453) -> (-9.6986, 3.9951) centre (-10.225, 4.8453) ccw
  arc A2 (-1.3634, 9.1558) -> (-1.358, 10.8529) centre (-1.8898, 10.0061) ccw
  arc A3 (1.5372, 8.6589) -> (0.4635, 8.6578) centre (1.0012, 7.8147) ccw
  arc A4 (8.5844, 2) -> (9.1204, 3.8442) centre (8.5844, 3) ccw
  arc A5 (-7.0853, 3.8431) -> (-6.5475, 2) centre (-6.5475, 3) ccw
  arc A6 (11.7503, 3.9899) -> (13.275, 4.8411) centre (12.275, 4.8411) ccw
  arc A7 (13.275, 15.2453) -> (11.7448, 16.0932) centre (12.275, 15.2453) ccw
  arc A8 (9.1204, 16.1558) -> (8.5844, 18) centre (8.5844, 17) ccw
  arc A9 (-6.5475, 18) -> (-7.0853, 16.1569) centre (-6.5475, 17) ccw
  arc A10 (0.4635, 11.3422) -> (1.5372, 11.3411) centre (1.0012, 12.1853) ccw
  arc A11 (3.3657, 10.854) -> (3.3712, 9.1548) centre (3.8959, 10.0061) ccw
  line L20 (-28.275, 20) -> (-28.275, 0)
  point P0 (-11.225, 17.05)
  point P1 (-11.225, 3.05)
  point P2 (13.275, 17.05)
  point P3 (13.275, 3.05)
  point P4 (-9.975, 18)
  point P5 (12.025, 18)
  point P6 (-9.975, 2)
  point P7 (12.025, 2)
  point P8 (1.025, 10.05)
  point P9 (1, 9)
  point P10 (0, 10)
  point P11 (1, 11)
  point P12 (2, 10)
  dimension "d77" = 3
  dimension "d78" = 17.05
  dimension "d79" = 2
  dimension "d80" = 2
  dimension "d81" = 11
  dimension "d82" = 7
  dimension "d83" = 22
  dimension "d84" = 22
  dimension "d85" = 14
  dimension "d86" = 14
  dimension "d87" = 4.25
  dimension "d88" = 3.05
  dimension "d89" = 1
  constraint perpendicular L6 L7
  constraint vertical L8
  constraint horizontal L10
  constraint perpendicular L7 L11
  constraint horizontal P0 P2
  constraint vertical P4 P6
  constraint coincident P0 L18
  constraint coincident P0 L7
  constraint tangent L18 A0
  constraint tangent L7 A0
  constraint coincident P1 L7
  constraint coincident P1 L19
  constraint tangent L7 A1
  constraint tangent L19 A1
  constraint equal A0 A1
  constraint tangent L19 A2
  constraint tangent L18 A2
  constraint equal A0 A2
  constraint tangent L12 A3
  constraint tangent L13 A3
  constraint equal A0 A3
  constraint coincident P7 L13
  constraint coincident P7 L11
  constraint tangent L13 A4
  constraint tangent L11 A4
  constraint equal A0 A4
  constraint coincident P6 L11
  constraint coincident P6 L12
  constraint tangent L11 A5
  constraint tangent L12 A5
  constraint equal A0 A5
  constraint coincident P3 L14
  constraint coincident P3 L8
  constraint tangent L14 A6
  constraint tangent L8 A6
  constraint equal A0 A6
  constraint coincident P2 L8
  constraint coincident P2 L15
  constraint tangent L8 A7
  constraint tangent L15 A7
  constraint equal A0 A7
  constraint coincident P5 L16
  constraint coincident P5 L10
  constraint tangent L16 A8
  constraint tangent L10 A8
  constraint equal A0 A8
  constraint coincident P4 L17
  constraint coincident P4 L10
  constraint tangent L17 A9
  constraint tangent L10 A9
  constraint equal A0 A9
  constraint tangent L16 A10
  constraint tangent L17 A10
  constraint equal A0 A10
  constraint tangent L14 A11
  constraint tangent L15 A11
  constraint equal A0 A11
  measures "d77" distance of L5 L8
  measures "d78" distance of L7 L9
  measures "d79" distance of L6 L10
  measures "d80" distance of L0 L11
  measures "d81" horizontal distance of P5 P8
  measures "d82" vertical distance of P2 P8
  measures "d83" distance of P4 P5
  measures "d84" distance of P6 P7
  measures "d85" distance of P2 P3
  measures "d86" distance of P0 P1
  measures "d87" distance of L5 P5
  measures "d88" distance of L0 P3
  measures "d89" radius of A0
extrude "Extrude8" cut sketch "Sketch10" against normal blind 65 contours L2 L3 L4 L8 L14 L15 A6 A7 A11 | L2 L3 L4 L8 | L7 L18 L19 A0 A1 A2 | L10 L16 L17 A8 A9 A10 | L11 L12 L13 A3 A4 A5
extrude "Extrude9" cut 2 faces at (27.0333, 28.275, 6.6667) (-23.5167, 28.275, 13.3333) along direction (0, -1, 0) blind 1.55
extrude "Extrude10" cut 1 faces at (-6.6667, 38.275, 13.3333) along direction (0, -1, 0) blind 4.5
fillet "Fillet4" radius 2.5 6 edges at (-20, 26.725, 10) (-20, 33.775, 10) (-30.55, 26.725, 10) (20, 33.775, 10) (20, 26.725, 10) (30.55, 26.725, 10)
sketch "Sketch11" plane through (0, 33.775, 0) normal (0, 1, 0) x (-1, 0, 0)
  line L0 (-17.5, 20) -> (-17.5, 0)
  line L1 (-17.5, 0) -> (17.5, 0)
  line L2 (17.5, 0) -> (17.5, 20)
  line L3 (17.5, 20) -> (-17.5, 20)
  line L4 (-22.5, 4.5) -> (22.5, 4.5)
  line L5 (22.5, 4.5) -> (22.5, 20)
  line L6 (22.5, 20) -> (-22.5, 20)
  line L7 (-22.5, 20) -> (-22.5, 4.5)
  dimension "d99" = 4.5
  dimension "d100" = 45
  dimension "d101" = 15.5
  dimension "d102" = 22.5
  constraint horizontal L4
  constraint vertical L5
  constraint horizontal L6
  constraint vertical L7
  measures "d99" distance of L1 L4
  measures "d100" distance of L5 L7
  measures "d101" distance of L4 L6
  measures "d102" distance of origin L7
extrude "Extrude11" cut sketch "Sketch11" against normal blind 7.05 contours L0 L2 L3 L4 L6 | L0 L4 L6 L7 | L2 L4 L5 L6
fillet "Fillet7" radius 2 1 edges at (0, 26.725, 4.5)
sketch "Sketch15" plane through (0, 26.725, 0) normal (0, 1, 0) x (-1, 0, 0)
  line L0 (-22.5, 0) -> (-22.5, 6.5)
  line L1 (-22.5, 6.5) -> (22.5, 6.5)
  line L2 (22.5, 6.5) -> (22.5, 0)
  line L3 (22.5, 0) -> (28.05, 0)
  line L4 (28.05, 0) -> (28.05, 20)
  line L5 (28.05, 20) -> (-28.05, 20)
  line L6 (-28.05, 20) -> (-28.05, 0)
  line L7 (-28.05, 0) -> (-22.5, 0)
  line L8 (22.5, 6.5) -> (-22.5, 6.5)
  line L9 (-22.5, 6.5) -> (-22.5, 0)
  line L10 (-22.5, 0) -> (22.5, 0)
  line L11 (22.5, 0) -> (22.5, 6.5)
  constraint horizontal L8
  constraint vertical L9
  constraint horizontal L10
  constraint vertical L11
  constraint coincident L0.start L7.end
  constraint coincident L1.end L2.start
extrude "Extrude15" cut sketch "Sketch15" along normal blind 15 contours L0 L1 L2 L8 L9 L10 L11
sketch "Sketch16" plane through (0, 0, 0) normal (0, 0, -1) x (1, 0, 0)
  circle A0 centre (24.05, -21.775) radius 1.5
  circle A1 centre (-24.05, -21.775) radius 1.5
  line L0 (-28.05, -26.725) -> (28.05, -26.725)
  arc A2 (28.05, -26.725) -> (30.55, -24.225) centre (28.05, -24.225) ccw
  line L1 (30.55, -24.225) -> (30.55, 16.275)
  line L2 (30.55, 16.275) -> (38.55, 16.275)
  line L3 (38.55, 16.275) -> (38.55, 26.275)
  line L4 (38.55, 26.275) -> (28.55, 26.275)
  line L5 (28.55, 26.275) -> (28.55, -14.525)
  arc A3 (26.05, -17.025) -> (28.55, -14.525) centre (26.05, -14.525) ccw
  line L6 (26.05, -17.025) -> (24.3, -17.025)
  arc A4 (24.3, -17.025) -> (19.3, -22.025) centre (24.3, -22.025) ccw
  line L7 (19.3, -22.025) -> (19.3, -23.775)
  arc A5 (16.8, -26.275) -> (19.3, -23.775) centre (16.8, -23.775) ccw
  line L8 (16.8, -26.275) -> (-16.8, -26.275)
  arc A6 (-19.3, -23.775) -> (-16.8, -26.275) centre (-16.8, -23.775) ccw
  line L9 (-19.3, -23.775) -> (-19.3, -22.025)
  arc A7 (-19.3, -22.025) -> (-24.3, -17.025) centre (-24.3, -22.025) ccw
  line L10 (-24.3, -17.025) -> (-26.05, -17.025)
  arc A8 (-28.55, -14.525) -> (-26.05, -17.025) centre (-26.05, -14.525) ccw
  line L11 (-28.55, -14.525) -> (-28.55, 26.275)
  line L12 (-28.55, 26.275) -> (-38.55, 26.275)
  line L13 (-38.55, 26.275) -> (-38.55, 16.275)
  line L14 (-38.55, 16.275) -> (-30.55, 16.275)
  line L15 (-30.55, 16.275) -> (-30.55, -24.225)
  arc A9 (-30.55, -24.225) -> (-28.05, -26.725) centre (-28.05, -24.225) ccw
  line L16 (25.55, -17.025) -> (24.3, -17.025)
  line L17 (-30.55, -22.025) -> (-30.55, -24.225)
  line L18 (-28.05, -26.725) -> (28.05, -26.725)
  line L19 (30.55, -24.225) -> (30.55, -22.025)
  line L20 (19.3, -23.775) -> (19.3, -22.025)
  line L21 (-19.3, -23.775) -> (-19.3, -22.025)
  arc A10 (28.05, -26.725) -> (30.55, -24.225) centre (28.05, -24.225) ccw
  arc A11 (-30.55, -24.225) -> (-28.05, -26.725) centre (-28.05, -24.225) ccw
  arc A12 (24.3, -17.025) -> (19.3, -22.025) centre (24.3, -22.025) ccw
  line L22 (-24.3, -17.025) -> (-25.55, -17.025)
  arc A13 (-19.3, -22.025) -> (-24.3, -17.025) centre (-24.3, -22.025) ccw
  line L23 (16.8, -26.275) -> (-16.8, -26.275)
  arc A14 (16.8, -26.275) -> (19.3, -23.775) centre (16.8, -23.775) ccw
  arc A15 (-19.3, -23.775) -> (-16.8, -26.275) centre (-16.8, -23.775) ccw
  circle A16 centre (24.05, -21.775) radius 1.5
  circle A17 centre (-24.05, -21.775) radius 1.5
  arc A18 (-25.55, -17.025) -> (-30.55, -22.025) centre (-25.55, -22.025) ccw
  arc A19 (30.55, -22.025) -> (25.55, -17.025) centre (25.55, -22.025) ccw
  dimension "d168" = 61.1
  dimension "d169" = 9.7
  dimension "d170" = 38.6
  dimension "d171" = 11.25
  dimension "d172" = 2.5
  dimension "d173" = 5
  dimension "d174" = 5
  dimension "d175" = 0.45
  dimension "d176" = 2.5
  dimension "d177" = 2.5
  dimension "d178" = 5
  dimension "d179" = 5
  constraint horizontal L16
  constraint vertical L17
  constraint horizontal L18
  constraint vertical L19
  constraint perpendicular L16 L20
  constraint perpendicular L16 L21
  constraint tangent L19 A10
  constraint tangent L18 A10
  constraint tangent L18 A11
  constraint tangent L17 A11
  constraint equal A10 A11
  constraint tangent L16 A12
  constraint tangent L20 A12
  constraint tangent L21 A13
  constraint tangent L22 A13
  constraint perpendicular L21 L23
  constraint tangent L23 A14
  constraint tangent L20 A14
  constraint tangent L21 A15
  constraint tangent L23 A15
  constraint concentric A0 A16
  constraint concentric A1 A17
  constraint tangent L22 A18
  constraint tangent L17 A18
  constraint tangent L19 A19
  constraint tangent L16 A19
  measures "d168" distance of L17 L19
  measures "d169" distance of L16 L18
  measures "d170" distance of L20 L21
  measures "d171" distance of L19 L20
  measures "d172" radius of A10
  measures "d173" radius of A12
  measures "d174" radius of A13
  measures "d175" distance of L18 L23
  measures "d176" radius of A14
  measures "d177" radius of A15
  measures "d178" radius of A18
  measures "d179" radius of A19
extrude "Extrude16" add sketch "Sketch16" along normal blind 20 contours L0 A2 L1 L6 A4 L7 A5 L8 A6 L9 A7 L10 L15 A9 L16 L17 L18 L19 L20 L21 A10 A11 A12 L22 A13 L23 A14 A15 A18 A19
sketch "Sketch18" plane through (0, 0, 20) normal (0, 0, 1) x (-1, 0, 0)
  line L0 (-28.05, -26.725) -> (28.05, -26.725)
  arc A0 (28.05, -26.725) -> (30.55, -24.225) centre (28.05, -24.225) ccw
  line L1 (30.55, -24.225) -> (30.55, 16.275)
  line L2 (30.55, 16.275) -> (40.55, 16.275)
  line L3 (40.55, 16.275) -> (40.55, 26.275)
  line L4 (40.55, 26.275) -> (28.55, 26.275)
  line L5 (28.55, 26.275) -> (28.55, -14.525)
  arc A1 (26.05, -17.025) -> (28.55, -14.525) centre (26.05, -14.525) ccw
  line L6 (26.05, -17.025) -> (24.3, -17.025)
  arc A2 (24.3, -17.025) -> (19.3, -22.025) centre (24.3, -22.025) ccw
  line L7 (19.3, -22.025) -> (19.3, -23.775)
  arc A3 (16.8, -26.275) -> (19.3, -23.775) centre (16.8, -23.775) ccw
  line L8 (16.8, -26.275) -> (-16.8, -26.275)
  arc A4 (-19.3, -23.775) -> (-16.8, -26.275) centre (-16.8, -23.775) ccw
  line L9 (-19.3, -23.775) -> (-19.3, -22.025)
  arc A5 (-19.3, -22.025) -> (-24.3, -17.025) centre (-24.3, -22.025) ccw
  line L10 (-24.3, -17.025) -> (-26.05, -17.025)
  arc A6 (-28.55, -14.525) -> (-26.05, -17.025) centre (-26.05, -14.525) ccw
  line L11 (-28.55, -14.525) -> (-28.55, 26.275)
  line L12 (-28.55, 26.275) -> (-40.55, 26.275)
  line L13 (-40.55, 26.275) -> (-40.55, 16.275)
  line L14 (-40.55, 16.275) -> (-30.55, 16.275)
  line L15 (-30.55, 16.275) -> (-30.55, -24.225)
  arc A7 (-30.55, -24.225) -> (-28.05, -26.725) centre (-28.05, -24.225) ccw
  circle A8 centre (24.05, -21.775) radius 1.5
  circle A9 centre (-24.05, -21.775) radius 1.5
  line L16 (19.3, -23.775) -> (-19.3, -23.775)
  line L17 (-19.3, -23.775) -> (-19.3, -26.725)
  line L18 (-19.3, -26.725) -> (19.3, -26.725)
  line L19 (19.3, -26.725) -> (19.3, -23.775)
  dimension "d192" = 2.95
  dimension "d193" = 38.6
  constraint horizontal L16
  constraint vertical L17
  constraint horizontal L18
  constraint vertical L19
  constraint coincident L7.end A3.end
  measures "d192" distance of L16 L18
  measures "d193" distance of L17 L19
extrude "Extrude17" cut sketch "Sketch18" against normal blind 10 contours L0 A3 L8 A4 L17 L18 L19